# Autodesk Inventor part: Bevel Gear1
Saved by Autodesk Inventor 2016 (Build 200138000, 138)
## iProperties
Created: 2016-07-28
Part Number: Bevel Gear1
Material: Steel, Mild
Document SubType Name: Modeling
Designer: Admin
Categories: <?xml version="1.0" encoding="UTF-16"?> <MemberInstance><Categories><FamilyTemplate><FamilyTemplateParameter ValueType="xs:double" Id="1" ObjectReferenceKey="da_z" ObjectType="kUserParameterObject"/><FamilyTemplateParameter ValueType="xs:double" Id="2" ObjectReferenceKey="da_b" ObjectType="kUserParameterObject"/><FamilyTemplateParameter ValueType="xs:double" Id="3" ObjectReferenceKey="da_beta" ObjectType="kUserParameterObject"/><FamilyTemplateParameter ValueType="xs:double" Id="4" ObjectReferenceKey="da_dae" ObjectType="kUserParameterObject"/><FamilyTemplateParameter ValueType="xs:double" Id="5" ObjectReferenceKey="da_ve" ObjectType="kUserParameterObject"/><FamilyTemplateParameter ValueType="xs:double" Id="6" ObjectReferenceKey="da_omega" ObjectType="kUserParameterObject"/><FamilyTemplateParameter ValueType="xs:string" Id="7" ObjectReferenceKey="EAIAABAAAAAAHwAAAAAAAIAAAAAAAAAA" ObjectType="83914240" SubObjectId="SurfaceGeometry"/></FamilyTemplate><ParamToTemplateMap><ParamToTemplate CategoryParameter="//CategoryParameter[@InternalName='046C89C9-8512-4d59-83FE-43B91F4F132A']" TemplateParameter="1"/><ParamToTemplate CategoryParameter="//CategoryParameter[@InternalName='2552DF32-E462-4b46-AEBF-C6C7768E72AC']" TemplateParameter="2"/><ParamToTemplate CategoryParameter="//CategoryParameter[@InternalName='C9EE641D-15FC-4fae-A226-E94C4372FDD7']" TemplateParameter="3"/><ParamToTemplate><ParamToTemplate CategoryParameter="//CategoryParameter[@InternalName='00B6519A-459B-49c7-AD84-2E56D39A5744']" ConstantValue="0.000000"/></ParamToTemplate><ParamToTemplate><ParamToTemplate CategoryParameter="//CategoryParameter[@InternalName='04B31F0E-C7A6-4894-AA32-9629BEFACF47']" ConstantValue="1.000000"/></ParamToTemplate><ParamToTemplate><ParamToTemplate CategoryParameter="//CategoryParameter[@InternalName='43CBEC2E-7847-49e7-A936-2F7889FCB2D9']" ConstantValue="0.200000"/></ParamToTemplate><ParamToTemplate><ParamToTemplate CategoryParameter="//CategoryParameter[@InternalName='B1EFC894-105D-4ebd-86BF-FA20ED196853']" ConstantValue="0.300000"/></ParamToTemplate><ParamToTemplate><ParamToTemplate CategoryParameter="//CategoryParameter[@InternalName='51175063-3D10-4879-93E8-6246FE8B403D']" ConstantValue="2060000000.000000"/></ParamToTemplate><ParamToTemplate><ParamToTemplate CategoryParameter="//CategoryParameter[@InternalName='A3A52E27-4454-46a9-B0BD-C932399B70AF']" ConstantValue="0.300000"/></ParamToTemplate><ParamToTemplate CategoryParameter="//CategoryParameter[@InternalName='2A200944-5A8C-41ca-B96E-8520D2E510F1']" TemplateParameter="4"/><ParamToTemplate><ParamToTemplate CategoryParameter="//CategoryParameter[@InternalName='1A637F62-92C8-44bc-B81F-10802510B579']" ConstantValue="4.238819"/></ParamToTemplate><ParamToTemplate CategoryParameter="//CategoryParameter[@InternalName='B52DD4BE-6863-48fb-BF58-89EF6F9EC65C']" TemplateParameter="5"/><ParamToTemplate><ParamToTemplate CategoryParameter="//CategoryParameter[@InternalName='3956BFF2-84D2-457d-93C2-9B0613DEBA67']" ConstantValue="9.989633"/></ParamToTemplate><ParamToTemplate CategoryParameter="//CategoryParameter[@InternalName='739CFA02-461B-4bf8-8049-181FCAD8B28F']" TemplateParameter="6"/><ParamToTemplate><ParamToTemplate CategoryParameter="//CategoryParameter[@InternalName='A27E999F-E2CE-4481-8A2A-EBF499C4C3C5']" ConstantValue="0.000000"/></ParamToTemplate><ParamToTemplate><ParamToTemplate CategoryParameter="//CategoryParameter[@InternalName='9E1B4470-B2D3-4ff1-B813-535BB4CDF51A']" ConstantValue="3520000.000000"/></ParamToTemplate><ParamToTemplate><ParamToTemplate CategoryParameter="//CategoryParameter[@InternalName='F8452263-BFF6-458c-9FB1-07C4B99E95CD']" ConstantValue="11400000.000000"/></ParamToTemplate><ParamToTemplate><ParamToTemplate CategoryParameter="//CategoryParameter[@InternalName='3E3BB259-FD49-497f-8171-6EBC954A3479']" ConstantValue="2.000000"/></ParamToTemplate><ParamToTemplate CategoryParameter="//CategoryParameter[@InternalName='27C3BAF2-7550-4e4b-AE2C-0DB134B7D9B7']" TemplateParameter="7"/></ParamToTemplateMap><Category DisplayName="Gear" InternalName="DC85795E-93AB-48d5-8EEE-5A27447B64BD" Mnemonic="Gear"><CategoryParameter DisplayName="z" InternalName="046C89C9-8512-4d59-83FE-43B91F4F132A" Mnemonic="z"/><CategoryParameter DisplayName="b" InternalName="2552DF32-E462-4b46-AEBF-C6C7768E72AC" Mnemonic="b"/><CategoryParameter DisplayName="||b|" InternalName="C9EE641D-15FC-4fae-A226-E94C4372FDD7" Mnemonic="beta"/><CategoryParameter DisplayName="x" InternalName="00B6519A-459B-49c7-AD84-2E56D39A5744" Mnemonic="x"/><CategoryParameter DisplayName="a*" InternalName="04B31F0E-C7A6-4894-AA32-9629BEFACF47" Mnemonic="a"/><CategoryParameter DisplayName="c*" InternalName="43CBEC2E-7847-49e7-A936-2F7889FCB2D9" Mnemonic="c"/><CategoryParameter DisplayName="r|.f|*" InternalName="B1EFC894-105D-4ebd-86BF-FA20ED196853" Mnemonic="rf"/><CategoryParameter DisplayName="E" InternalName="51175063-3D10-4879-93E8-6246FE8B403D" Mnemonic="E"/><CategoryParameter DisplayName="||m|" InternalName="A3A52E27-4454-46a9-B0BD-C932399B70AF" Mnemonic="mi"/><Category DisplayName="BevelGear" InternalName="0C98F69A-0C2B-4791-B2FE-7691BB227E77" Mnemonic="BevelGear"><CategoryParameter DisplayName="d|.ae|" InternalName="2A200944-5A8C-41ca-B96E-8520D2E510F1" Mnemonic="dae"/><CategoryParameter DisplayName="d|.ai|" InternalName="1A637F62-92C8-44bc-B81F-10802510B579" Mnemonic="dai"/><CategoryParameter DisplayName="A|.e|" InternalName="B52DD4BE-6863-48fb-BF58-89EF6F9EC65C" Mnemonic="ve"/><CategoryParameter DisplayName="A|.i|" InternalName="3956BFF2-84D2-457d-93C2-9B0613DEBA67" Mnemonic="vi"/><CategoryParameter DisplayName="||S|" InternalName="739CFA02-461B-4bf8-8049-181FCAD8B28F" Mnemonic="omega"/><CategoryParameter DisplayName="x|.t|" InternalName="A27E999F-E2CE-4481-8A2A-EBF499C4C3C5" Mnemonic="xt"/><CategoryParameter DisplayName="||s||.Flim|" InternalName="9E1B4470-B2D3-4ff1-B813-535BB4CDF51A" Mnemonic="sFlim"/><CategoryParameter DisplayName="||s||.Hlim|" InternalName="F8452263-BFF6-458c-9FB1-07C4B99E95CD" Mnemonic="sHlim"/><CategoryParameter DisplayName="type" InternalName="3E3BB259-FD49-497f-8171-6EBC954A3479" Mnemonic="type"/><CategoryParameter DisplayName="PitchDiameter" InternalName="27C3BAF2-7550-4e4b-AE2C-0DB134B7D9B7" Mnemonic="IDS_PITCHDIAM"/></Category></Category></Categories></MemberInstance>
Mass: 60.9118 g
Surface Area: 34.3074 cm^2
Volume: 7.7496 cm^3
Density: 7.86 g/cm^3
Appearance: Steel
CustomPartVersion: 1
Author: Admin
Autodesk Inventor part; units mm, degrees
ref_plane "Mesh Plane2" through (0, 0, 0) normal (0.9781476, 0.2079117, 0) x (0, 0, 1)
sketch "Teeth Body Sketch" plane through (0, 0, 0) normal (1, 0, 0) x (0, 1, 0)
  line L0 (0, 0) -> (18.96166, -120.663439) construction
  line L1 (18.96166, -120.663439) -> (25.346087, -119.466359)
  line L2 (25.346087, -119.466359) -> (0, 0) construction
  line L3 (22.5, -120) -> (0, 0) construction
  line L4 (15.855512, -100.897316) -> (21.194093, -99.896332)
  line L5 (18.96166, -120.663439) -> (15.855512, -100.897316)
  line L6 (25.346087, -119.466359) -> (21.194093, -99.896332)
  line L7 (0, -39.386751) -> (0, 6.564458)
  line L8 (0, -120) -> (25.346087, -120) construction
  dimension "d0" = 45
  dimension "d1" = 37.92332
  dimension "d2" = 50.69217
  dimension "d3" = 20
  dimension "d4" = 119.46636
  constraints: 16 end point, 4 point on line, 3 perpendicular, 2 collinear, 1 horizontal alignment, 1 vertical alignment
  measures "d0" diameter of L3.start L7
  measures "d1" diameter of L0.end L7
  measures "d2" diameter of L1.end L7
  measures "d3" distance between parallel lines of L1 L4
  measures "d4" vertical distance of L1.end L0.start
revolve "Teeth Body" add sketch "Teeth Body Sketch" angle 360 about axis through (0, 0, 0) along (0, 0, 1)
ref_plane "Tooth Plane" through (0, 22.5, -120) normal (0, -0.1842885, 0.9828722) x (1, 0, 0)
sketch "Start Sketch" plane through (0, 22.5, -120) normal (0, -0.1842885, 0.9828722) x (1, 0, 0)
  line L0 (0, -23.505131) -> (0, 10.644758)
  arc A0 (-1.448073, -4.379482) -> (-6.849403, 3.985372) centre (-10.10213, -4.041262) ccw
  arc A1 (6.849403, 3.985372) -> (1.448073, -4.379482) centre (10.10213, -4.041262) ccw
  line L1 (-1.448073, -4.379482) -> (1.448073, -4.379482)
  arc A2 (6.849403, 3.985372) -> (-6.849403, 3.985372) centre (0, -22.892091) ccw
  dimension "d7" = 8.66066
  dimension "d8" = 10.10213
  dimension "d9" = 18.85083
  dimension "d57" = 27.73648
  dimension "d58" = 18.51261
  constraints: 6 point on circle, 3 centre point, 3 symmetric about line, 2 end point, 1 coincident, 1 perpendicular, 1 other
  measures "d7" radius of A0
  measures "d8" horizontal distance of point (0, -22.892) A0.centre
  measures "d9" vertical distance of point (0, -22.892) A0.centre
  measures "d57" radius of A2
  measures "d58" distance from line of A2.centre L1
sketch "End Sketch" plane through (0, 18.754375, -100.023335) normal (0, -0.1842885, 0.9828722) x (1, 0, 0)
  line L0 (0, -15.358918) -> (0, 6.982715)
  arc A0 (-1.208458, -3.631907) -> (-5.716017, 3.348795) centre (-8.430508, -3.349654) ccw
  arc A1 (5.716017, 3.348795) -> (1.208458, -3.631907) centre (8.430508, -3.349654) ccw
  line L1 (-1.208458, -3.631907) -> (1.208458, -3.631907)
  arc A2 (5.716017, 3.348795) -> (-5.716017, 3.348795) centre (0, -19.081194) ccw
  dimension "d12" = 7.22756
  dimension "d15" = 8.43051
  dimension "d16" = 15.73154
  dimension "d59" = 23.14686
  dimension "d60" = 15.44929
  constraints: 6 point on circle, 3 centre point, 3 symmetric about line, 2 end point, 1 coincident, 1 other
  measures "d12" radius of A0
  measures "d15" horizontal distance of A0.centre point (0, -19.081)
  measures "d16" vertical distance of A0.centre point (0, -19.081)
  measures "d59" radius of A2
  measures "d60" distance from line of A2.centre L1
loft "Loft" cut profiles "Start Sketch", "End Sketch"
pattern_circular "Circular Pattern" count 15 over 360 about axis through (0, 0, 0) along (0, 0, 1) of "Loft"
ref_plane "End Plane" through (0, 18.754375, -100.023335) normal (0, -0.1842885, 0.9828722) x (1, 0, 0)
sketch3d "3D Sketch Right"
ref_plane "End Plane Right" through (-6.57358, 17.564585, -100.023335) normal (0.0645948, -0.1725971, 0.9828722) x (0.9365593, 0.3505092, 0)
sketch "End Sketch Right" plane through (-6.57358, 17.564585, -100.023335) normal (0.0645948, -0.1725971, 0.9828722) x (0.9365593, 0.3505092, 0)
  arc A0 (-1.208458, -3.631907) -> (-5.716017, 3.348795) centre (-8.430508, -3.349654) ccw
  line L0 (0, -29.61696) -> (0, 14.326813)
  arc A1 (5.716017, 3.348795) -> (1.208458, -3.631907) centre (8.430508, -3.349654) ccw
  line L1 (-1.208458, -3.631907) -> (1.208458, -3.631907)
  arc A2 (5.716017, 3.348795) -> (-5.716017, 3.348795) centre (0, -19.081194) ccw
  dimension "d70" = 8.43051
  dimension "d71" = 15.73154
  dimension "d72" = 7.22756
  dimension "d73" = 15.44929
  dimension "d74" = 23.14686
  constraints: 6 point on circle, 3 centre point, 3 symmetric about line, 2 end point, 1 coincident, 1 perpendicular, 1 other
  measures "d70" horizontal distance of A2.centre A0.centre
  measures "d71" vertical distance of point (0, -19.081) A0.centre
  measures "d72" radius of A0
  measures "d73" distance from line of point (0, -19.081) L1
  measures "d74" radius of A2
feature "Loft Right" [suppressed]
pattern_circular "Circular Pattern Right" [suppressed]
sketch3d "3D Sketch Left"
ref_plane "End Plane Left" through (6.547167, 17.564585, -100.014663) normal (-0.0643417, -0.1726145, 0.9828857) x (0.937021, -0.3492729, 0)
sketch "End Sketch Left" plane through (6.547167, 17.564585, -100.014663) normal (-0.0643417, -0.1726145, 0.9828857) x (0.937021, -0.3492729, 0)
  line L0 (0, -37.55195) -> (0, 20.553619)
  arc A0 (-1.208458, -3.624421) -> (-5.716017, 3.356282) centre (-8.430508, -3.342168) ccw
  arc A1 (5.716017, 3.356282) -> (1.208458, -3.624421) centre (8.430508, -3.342168) ccw
  line L1 (-1.208458, -3.624421) -> (1.208458, -3.624421)
  ellipse E0 centre (0, -18.402526) end of major axis (21.194093, -18.402526) minor radius 20.831372
  arc A2 (5.716017, 3.356282) -> (-5.716017, 3.356282) centre (0, -19.073708) ccw
  dimension "d56" = 20.83137
  dimension "d30" = 7.22756
  dimension "d31" = 8.43051
  dimension "d32" = 15.73154
  dimension "d61" = 23.14686
  dimension "d62" = 15.44929
  constraints: 6 point on circle, 3 centre point, 3 symmetric about line, 2 end point, 1 coincident, 2 other
  measures "d30" radius of A0
  measures "d31" horizontal distance of point (0, -19.074) A0.centre
  measures "d32" vertical distance of A0.centre point (0, -19.074)
  measures "d61" radius of A2
  measures "d62" distance from line of point (0, -19.074) L1
feature "Loft Left" [suppressed]
pattern_circular "Circular Pattern Left" [suppressed]
sketch "Body Sketch" plane through (0, 0, 0) normal (1, 0, 0) x (0, 1, 0)
  line L0 (0, -35.037536) -> (0, -19.530831)
  line L1 (18.96166, -120.663439) -> (15.855512, -100.897316)
  line L2 (15.855512, -100.897316) -> (0, -100.897316)
  line L3 (18.96166, -120.663439) -> (0, -120.663439)
  constraints: 4 end point, 2 perpendicular, 2 point on line
sketch "Body Sketch outline for Fix Body" plane through (0, 0, 0) normal (1, 0, 0) x (0, 1, 0)
  line L0 (0, -120.663439) -> (18.96166, -120.663439)
  line L1 (0, -100.897316) -> (0, -120.663439)
  line L2 (15.855512, -100.897316) -> (0, -100.897316)
  line L3 (18.96166, -120.663439) -> (15.855512, -100.897316)
revolve "Fix Body" add sketch "Body Sketch outline for Fix Body" angle 360 about axis through (0, 0, 0) along (0, 0, 1)
sketch "Sketch6" plane through (0, 0, 0) normal (1, 0, 0) x (0, 1, 0)
  line L0 (22.5, -120) -> (0, 0)
  line L1 (0, -37.799919) -> (0, 6.299986)
surface revolve "Pitch Diameter" sketch "Sketch6" angle 360 about axis through (0, 0, 0) along (0, 0, 1) shown no curves L0
equation "\"d0\" = da_de"
equation "\"d1\" = da_dfe"
equation "\"d2\" = da_dae"
equation "\"d3\" = da_b"
equation "\"d4\" = da_ve"
equation "\"d7\" = fd_rr"
equation "\"d8\" = fd_x"
equation "\"d9\" = fd_y"
equation "\"d57\" = 0.5 * fd_dva + 0.3 * da_he"
equation "\"d58\" = 0.5 * fd_dva - 1.12 * da_he"
equation "\"da_teethtype\" = 0"
equation "\"da_b\" = 20"
equation "\"da_de\" = 45"
equation "\"da_dae\" = 50.69217"
equation "\"da_dfe\" = 37.92332"
equation "\"da_le\" = 122.09115"
equation "\"da_omega\" = 90deg"
equation "\"da_beta\" = 0"
equation "\"da_delta\" = 10.619655deg"
equation "\"da_alpha\" = 20deg"
equation "\"da_he\" = 6.49568"
equation "\"da_ve\" = 119.46636"
equation "\"da_zv\" = 15.261394"
equation "\"fd_loft\" = da_b + 0.05 * da_he"
equation "\"fd_x\" = fd_x1 + fd_x2"
equation "\"fd_y\" = fd_y1 - fd_y2"
equation "\"fd_dd\" = fd_dva - 0.8 * da_he"
equation "\"da_dvw\" = 45.78418"
equation "\"d11\" = fd_loft"
equation "\"da_dm\" = 41.31423"
equation "\"da_x\" = 0"
equation "\"da_m\" = 3"
equation "\"d50\" = da_omega"
equation "\"fd_rr\" = 8.660663"
equation "\"fd_dva\" = 51.57555"
equation "\"fd_x1\" = 2.378076"
equation "\"fd_x2\" = 7.724054"
equation "\"fd_y1\" = 22.768237"
equation "\"fd_y2\" = 3.917408"
body "Solid1"
body "Srf1"
